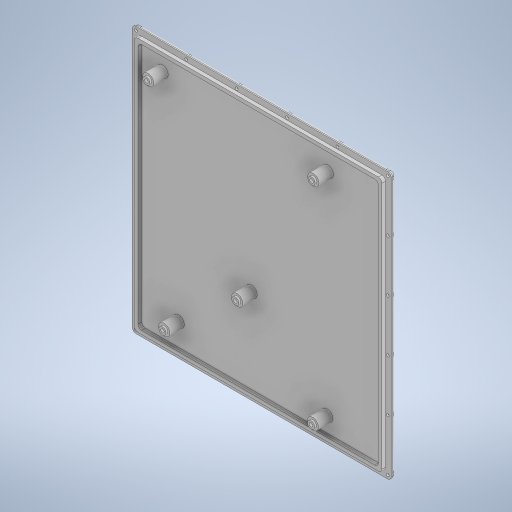
# Autodesk Inventor part: bottom
Saved by Autodesk Inventor 2024 (Build 280153000, 153)
## iProperties
Created: 2023-05-26
Part Number: bottom
Material: Generic
Document SubType Name: Modeling
Designer: elect
Density: 1 g/cm^3
Appearance: Default
Author: elect
Autodesk Inventor part; units mm, degrees
ref_plane "YZ Plane" through (0, 0, 0) normal (1, 0, 0) x (0, 1, 0)
ref_plane "XZ Plane" through (0, 0, 0) normal (0, 1, 0) x (-1, 0, 0)
ref_plane "XY Plane" through (0, 0, 0) normal (0, 0, 1) x (1, 0, 0)
sketch "Sketch1" plane through (0, 0, 0) normal (0, 0, 1) x (1, 0, 0)
  line L0 (-95.0021, 142.819) -> (127.2479, 142.819)
  line L1 (130.4229, 139.644) -> (130.4229, -88.956)
  line L2 (127.2479, -92.131) -> (-95.0021, -92.131)
  line L3 (-98.1771, -88.956) -> (-98.1771, 139.644)
  arc A0 (-95.0021, 142.819) -> (-98.1771, 139.644) centre (-95.0021, 139.644) ccw
  arc A1 (-98.1771, -88.956) -> (-95.0021, -92.131) centre (-95.0021, -88.956) ccw
  arc A2 (127.2479, -92.131) -> (130.4229, -88.956) centre (127.2479, -88.956) ccw
  arc A3 (130.4229, 139.644) -> (127.2479, 142.819) centre (127.2479, 139.644) ccw
  point P0 (0, 0)
  point P1 (130.4229, -92.131)
  point P2 (130.4229, 142.819)
  point P3 (-98.1771, -92.131)
  dimension "d0" = 228.6
  dimension "d1" = 234.95
  dimension "d2" = 3.175
  constraints: 8 end point, 8 point on circle, 8 tangent, 6 point on line, 4 centre point, 3 equal radius, 2 parallel, 1 horizontal, 1 perpendicular
  measures "d0" distance of point (130.423, -92.131) point (-98.177, -92.131)
  measures "d1" distance of point (130.423, 142.819) point (130.423, -92.131)
  measures "d2" radius of A0
extrude "Extrusion1" add sketch "Sketch1" along normal blind 4.064
sketch "Sketch2" plane through (0, 0, 0) normal (0, 0, -1) x (-1, 0, 0)
  circle A0 centre (-105.0229, 117.419) radius 6.477
  circle A1 centre (72.7771, 117.419) radius 6.477
  circle A2 centre (72.7771, -66.731) radius 6.477
  circle A3 centre (-105.0229, -66.731) radius 6.477
  line L0 (-130.4229, -88.956) -> (-130.4229, 139.644) projected
  line L1 (98.1771, 139.644) -> (98.1771, -88.956) projected
  line L2 (95.0021, -92.131) -> (-127.2479, -92.131) projected
  line L3 (-127.2479, 142.819) -> (95.0021, 142.819) projected
  point P0 (0, 0)
  dimension "d18" = 3.175
  dimension "d19" = 3.175
  dimension "d5" = 12.954
  dimension "d6" = 25.4
  dimension "d7" = 25.4
  dimension "d8" = 25.4
  dimension "d9" = 25.4
  constraints: 4 centre point, 3 equal radius, 2 horizontal alignment, 2 vertical alignment
  measures "d5" diameter of A0
  measures "d6" distance from line of L0 A0.centre
  measures "d7" distance from line of L1 A1.centre
  measures "d8" distance from line of L2 A2.centre
  measures "d9" distance from line of L3 A0.centre
extrude "Extrusion2" cut sketch "Sketch2" against normal blind 2.032
sketch "Sketch3" plane through (0, 0, 4.064) normal (0, 0, 1) x (1, 0, 0)
  line L0 (-89.9221, 137.739) -> (122.1679, 137.739)
  line L1 (125.3429, 134.564) -> (125.3429, -83.876)
  line L2 (122.1679, -87.051) -> (-89.9221, -87.051)
  line L3 (-93.0971, -83.876) -> (-93.0971, 134.564)
  line L4 (127.2479, 142.819) -> (-95.0021, 142.819) projected
  line L5 (-95.0021, -92.131) -> (127.2479, -92.131) projected
  line L6 (130.4229, -88.956) -> (130.4229, 139.644) projected
  line L7 (-98.1771, 139.644) -> (-98.1771, -88.956) projected
  arc A0 (-89.9221, 137.739) -> (-93.0971, 134.564) centre (-89.9221, 134.564) ccw
  arc A1 (125.3429, 134.564) -> (122.1679, 137.739) centre (122.1679, 134.564) ccw
  arc A2 (122.1679, -87.051) -> (125.3429, -83.876) centre (122.1679, -83.876) ccw
  arc A3 (-93.0971, -83.876) -> (-89.9221, -87.051) centre (-89.9221, -83.876) ccw
  line L8 (-86.7471, 134.564) -> (118.9929, 134.564)
  line L9 (122.1679, 131.389) -> (122.1679, -80.701)
  line L10 (118.9929, -83.876) -> (-86.7471, -83.876)
  line L11 (-89.9221, -80.701) -> (-89.9221, 131.389)
  arc A4 (-86.7471, 134.564) -> (-89.9221, 131.389) centre (-86.7471, 131.389) ccw
  arc A5 (122.1679, 131.389) -> (118.9929, 134.564) centre (118.9929, 131.389) ccw
  arc A6 (118.9929, -83.876) -> (122.1679, -80.701) centre (118.9929, -80.701) ccw
  arc A7 (-89.9221, -80.701) -> (-86.7471, -83.876) centre (-86.7471, -80.701) ccw
  point P0 (0, 0)
  point P1 (-93.0971, 25.344)
  dimension "d12" = 5.08
  dimension "d13" = 5.08
  dimension "d14" = 5.08
  dimension "d15" = 5.08
  dimension "d16" = 3.175
  dimension "d17" = 3.175
  dimension "d18" = 3.175
  dimension "d19" = 3.175
  dimension "d20" = 3.175
  dimension "d21" = 3.175
  constraints: 16 end point, 16 point on circle, 16 tangent, 8 centre point, 6 equal radius, 4 parallel, 2 horizontal, 2 perpendicular, 2 point on line, 1 midpoint
  measures "d12" distance between parallel lines of L4 L0
  measures "d13" distance between parallel lines of L5 L2
  measures "d14" distance between parallel lines of L6 L1
  measures "d15" distance between parallel lines of L7 L3
  measures "d16" radius of A0
  measures "d17" distance between parallel lines of L0 L8
  measures "d18" distance between parallel lines of L1 L9
  measures "d19" distance between parallel lines of L2 L10
  measures "d20" distance from line of L11 point (-93.097, 25.344)
  measures "d21" radius of A4
extrude "Extrusion3" add sketch "Sketch3" along normal blind 3.175
sketch "Sketch5" plane through (0, 0, 4.064) normal (0, 0, 1) x (1, 0, 0)
  circle A0 centre (-57.2421, -63.896) radius 5
  circle A1 centre (73.8473, -70.2206) radius 5
  circle A2 centre (7.0453, -9.0066) radius 5
  arc A3 (-89.9221, -80.701) -> (-86.7471, -83.876) centre (-86.7471, -80.701) ccw projected
  circle A4 centre (-71.4661, 120) radius 5
  circle A5 centre (74.3553, 116.4694) radius 5
  point P0 (0, 0)
  point P1 (-88.9921, -82.946)
  point P2 (-88.9921, -82.946)
  dimension "d62" = 6.3246
  dimension "d63" = 54.8894
  dimension "d64" = 64.2874
  dimension "d65" = 10
  dimension "d66" = 31.75
  dimension "d67" = 19.05
  dimension "d68" = 183.896
  dimension "d69" = 14.224
  dimension "d70" = 180.3654
  dimension "d84" = 131.0894
  dimension "d85" = 131.5974
  constraints: 5 centre point, 4 equal radius, 2 point on circle
  measures "d62" vertical distance of A0.centre A1.centre
  measures "d63" vertical distance of A2.centre A0.centre
  measures "d64" horizontal distance of A2.centre A0.centre
  measures "d65" diameter of A0
  measures "d66" horizontal distance of point (-88.992, -82.946) A0.centre
  measures "d67" vertical distance of point (-88.992, -82.946) A0.centre
  measures "d68" vertical distance of A0.centre A4.centre
  measures "d69" horizontal distance of A0.centre A4.centre
  measures "d70" vertical distance of A5.centre A0.centre
  measures "d84" horizontal distance of A1.centre A0.centre
  measures "d85" horizontal distance of A5.centre A0.centre
extrude "Extrusion4" add sketch "Sketch5" along normal blind 12.7
sketch "Sketch6" plane through (7.0453, -9.0066, 16.764) normal (0, 0, 1) x (1, 0, 0)
  circle A0 centre (0, 0) radius 3.2
  circle A1 centre (-64.2874, -54.8894) radius 5 projected
  circle A2 centre (-64.2874, -54.8894) radius 3.2
  circle A3 centre (66.802, -61.214) radius 5 projected
  circle A4 centre (66.802, -61.214) radius 3.2
  circle A5 centre (67.31, 125.476) radius 5 projected
  circle A6 centre (67.31, 125.476) radius 3.2
  circle A7 centre (-78.5114, 129.0066) radius 5 projected
  circle A8 centre (-78.5114, 129.0066) radius 3.2
  point P0 (-7.0453, 9.0066)
  point P1 (70.9479, -62.1693)
  point P2 (61.1321, -62.1693)
  dimension "d74" = 6.4
  constraints: 5 centre point, 4 coincident, 4 equal radius, 1 other
  measures "d74" diameter of A8
extrude "Extrusion5" add sketch "Sketch6" along normal blind 1.6383 contours A0 | A2 | A4 | A6 | A8
sketch "Sketch7" plane through (7.0453, -9.0066, 18.4023) normal (0, 0, 1) x (1, 0, 0)
  circle A0 centre (-78.5114, 129.0066) radius 3.2 projected
  circle A1 centre (67.31, 125.476) radius 3.2 projected
  circle A2 centre (0, 0) radius 3.2 projected
  circle A3 centre (-64.2874, -54.8894) radius 3.2 projected
  circle A4 centre (66.802, -61.214) radius 3.2 projected
  point P0 (-7.0453, 9.0066)
  constraints: 5 coincident
hole "Hole2" at (-71.4661, 120, 18.4023) at (74.3553, 116.4694, 18.4023) at (-57.2421, -63.896, 18.4023) at (73.8473, -70.2206, 18.4023) at (7.0453, -9.0066, 18.4023) direction (0, 0, -1) diameter 3.175 depth 7.62 tip angle 118
sketch "Sketch11" plane through (0, 0, 0) normal (0, 0, -1) x (-1, 0, 0)
  arc A0 (-127.2479, 142.819) -> (-130.4229, 139.644) centre (-127.2479, 139.644) ccw projected
  line L0 (89.9221, 137.739) -> (-122.1679, 137.739) projected
  line L1 (-125.3429, 134.564) -> (-125.3429, -83.876) projected
  point P0 (0, 0)
  point P1 (-82.7979, 139.644)
  point P2 (-38.3479, 139.644)
  point P3 (6.1021, 139.644)
  point P4 (50.5521, 139.644)
  point P5 (95.0021, 139.644)
  point P6 (-127.2479, 93.924)
  point P7 (-127.2479, 48.204)
  point P8 (-127.2479, 2.484)
  point P9 (-127.2479, -43.236)
  point P10 (-127.2479, -88.956)
  point P11 (-82.7979, -88.956)
  point P12 (-38.3479, -88.956)
  point P13 (6.1021, -88.956)
  point P14 (50.5521, -88.956)
  point P15 (95.0021, -88.956)
  point P16 (95.0021, -43.236)
  point P17 (95.0021, 2.484)
  point P18 (95.0021, 48.204)
  point P19 (95.0021, 93.924)
  dimension "d124" = 44.45
  dimension "d131" = 45.72
  dimension "d138" = 44.45
  dimension "d145" = 45.72
  constraints: 2 horizontal, 2 vertical, 1 coincident, 19 other
  measures "d124" distance of point (-127.248, 139.644) point (-82.798, 139.644)
  measures "d131" distance of point (-127.248, 139.644) point (-127.248, 93.924)
  measures "d138" distance of point (-127.248, -88.956) point (-82.798, -88.956)
  measures "d145" distance of point (95.002, -88.956) point (95.002, -43.236)
hole "Hole4" at (127.2479, 139.644, 0) at (82.7979, 139.644, 0) at (38.3479, 139.644, 0) at (-6.1021, 139.644, 0) at (-50.5521, 139.644, 0) at (-95.0021, 139.644, 0) at (127.2479, 93.924, 0) at (127.2479, 48.204, 0) at (127.2479, 2.484, 0) at (127.2479, -43.236, 0) at (127.2479, -88.956, 0) at (82.7979, -88.956, 0) at (38.3479, -88.956, 0) at (-6.1021, -88.956, 0) at (-50.5521, -88.956, 0) at (-95.0021, -88.956, 0) at (-95.0021, -43.236, 0) at (-95.0021, 2.484, 0) at (-95.0021, 48.204, 0) at (-95.0021, 93.924, 0) direction (0, 0, 1) diameter 2.54 end through all counterbore diameter 5.08 counterbore depth 2.54
fillet "Fillet3" radius 3.048 8 edges at (-97.2471, 141.8891, 0) (-98.1771, 25.344, 0) (-97.2471, -91.201, 0) (16.1229, -92.131, 0) (129.493, -91.201, 0) (130.4229, 25.344, 0) (129.493, 141.8891, 0) (16.1229, 142.819, 0)
body "Solid1"
